Autodesk Inventor part; units mm, degrees
(part 5 of 6)
  line L3785 (22.09, 25.7636) -> (22.09, 26.7636)
  line L3786 (22.09, 26.7636) -> (21.09, 26.7636)
  line L3787 (21.09, 26.7636) -> (21.09, 25.7636)
  line L3788 (21.9917, 25.7636) -> (22.9917, 25.7636)
  line L3789 (22.9917, 25.7636) -> (22.9917, 26.7636)
  line L3790 (22.9917, 26.7636) -> (21.9917, 26.7636)
  line L3791 (21.9917, 26.7636) -> (21.9917, 25.7636)
  line L3792 (12.7334, 25.789) -> (13.7334, 25.789)
  line L3793 (13.7334, 25.789) -> (13.7334, 26.789)
  line L3794 (13.7334, 26.789) -> (12.7334, 26.789)
  line L3795 (12.7334, 26.789) -> (12.7334, 25.789)
  line L3796 (14.4479, 25.789) -> (15.4479, 25.789)
  line L3797 (15.4479, 25.789) -> (15.4479, 26.789)
  line L3798 (15.4479, 26.789) -> (14.4479, 26.789)
  line L3799 (14.4479, 26.789) -> (14.4479, 25.789)
  line L3800 (15.0321, 25.789) -> (16.0321, 25.789)
  line L3801 (16.0321, 25.789) -> (16.0321, 26.789)
  line L3802 (16.0321, 26.789) -> (15.0321, 26.789)
  line L3803 (15.0321, 26.789) -> (15.0321, 25.789)
  line L3804 (19.4517, 25.789) -> (20.4517, 25.789)
  line L3805 (20.4517, 25.789) -> (20.4517, 26.789)
  line L3806 (20.4517, 26.789) -> (19.4517, 26.789)
  line L3807 (19.4517, 26.789) -> (19.4517, 25.789)
  line L3808 (20.3661, 25.789) -> (21.3661, 25.789)
  line L3809 (21.3661, 25.789) -> (21.3661, 26.789)
  line L3810 (21.3661, 26.789) -> (20.3661, 26.789)
  line L3811 (20.3661, 26.789) -> (20.3661, 25.789)
  line L3812 (21.0773, 25.789) -> (22.0773, 25.789)
  line L3813 (22.0773, 25.789) -> (22.0773, 26.789)
  line L3814 (22.0773, 26.789) -> (21.0773, 26.789)
  line L3815 (21.0773, 26.789) -> (21.0773, 25.789)
  line L3816 (22.0171, 25.789) -> (23.0171, 25.789)
  line L3817 (23.0171, 25.789) -> (23.0171, 26.789)
  line L3818 (23.0171, 26.789) -> (22.0171, 26.789)
  line L3819 (22.0171, 26.789) -> (22.0171, 25.789)
  line L3820 (12.7588, 25.8144) -> (13.7588, 25.8144)
  line L3821 (13.7588, 25.8144) -> (13.7588, 26.8144)
  line L3822 (13.7588, 26.8144) -> (12.7588, 26.8144)
  line L3823 (12.7588, 26.8144) -> (12.7588, 25.8144)
  line L3824 (14.4733, 25.8144) -> (15.4733, 25.8144)
  line L3825 (15.4733, 25.8144) -> (15.4733, 26.8144)
  line L3826 (15.4733, 26.8144) -> (14.4733, 26.8144)
  line L3827 (14.4733, 26.8144) -> (14.4733, 25.8144)
  line L3828 (19.4517, 25.8144) -> (20.4517, 25.8144)
  line L3829 (20.4517, 25.8144) -> (20.4517, 26.8144)
  line L3830 (20.4517, 26.8144) -> (19.4517, 26.8144)
  line L3831 (19.4517, 26.8144) -> (19.4517, 25.8144)
  line L3832 (20.3661, 25.8144) -> (21.3661, 25.8144)
  line L3833 (21.3661, 25.8144) -> (21.3661, 26.8144)
  line L3834 (21.3661, 26.8144) -> (20.3661, 26.8144)
  line L3835 (20.3661, 26.8144) -> (20.3661, 25.8144)
  line L3836 (21.0773, 25.8144) -> (22.0773, 25.8144)
  line L3837 (22.0773, 25.8144) -> (22.0773, 26.8144)
  line L3838 (22.0773, 26.8144) -> (21.0773, 26.8144)
  line L3839 (21.0773, 26.8144) -> (21.0773, 25.8144)
  line L3840 (22.0171, 25.8144) -> (23.0171, 25.8144)
  line L3841 (23.0171, 25.8144) -> (23.0171, 26.8144)
  line L3842 (23.0171, 26.8144) -> (22.0171, 26.8144)
  line L3843 (22.0171, 26.8144) -> (22.0171, 25.8144)
  line L3844 (12.7715, 25.8398) -> (13.7715, 25.8398)
  line L3845 (13.7715, 25.8398) -> (13.7715, 26.8398)
  line L3846 (13.7715, 26.8398) -> (12.7715, 26.8398)
  line L3847 (12.7715, 26.8398) -> (12.7715, 25.8398)
  line L3848 (14.4987, 25.8398) -> (15.4987, 25.8398)
  line L3849 (15.4987, 25.8398) -> (15.4987, 26.8398)
  line L3850 (15.4987, 26.8398) -> (14.4987, 26.8398)
  line L3851 (14.4987, 26.8398) -> (14.4987, 25.8398)
  line L3852 (19.4517, 25.8398) -> (20.4517, 25.8398)
  line L3853 (20.4517, 25.8398) -> (20.4517, 26.8398)
  line L3854 (20.4517, 26.8398) -> (19.4517, 26.8398)
  line L3855 (19.4517, 26.8398) -> (19.4517, 25.8398)
  line L3856 (20.3788, 25.8398) -> (21.3788, 25.8398)
  line L3857 (21.3788, 25.8398) -> (21.3788, 26.8398)
  line L3858 (21.3788, 26.8398) -> (20.3788, 26.8398)
  line L3859 (20.3788, 26.8398) -> (20.3788, 25.8398)
  line L3860 (21.0519, 25.8398) -> (22.0519, 25.8398)
  line L3861 (22.0519, 25.8398) -> (22.0519, 26.8398)
  line L3862 (22.0519, 26.8398) -> (21.0519, 26.8398)
  line L3863 (21.0519, 26.8398) -> (21.0519, 25.8398)
  line L3864 (22.0425, 25.8398) -> (23.0425, 25.8398)
  line L3865 (23.0425, 25.8398) -> (23.0425, 26.8398)
  line L3866 (23.0425, 26.8398) -> (22.0425, 26.8398)
  line L3867 (22.0425, 26.8398) -> (22.0425, 25.8398)
  line L3868 (12.7969, 25.8652) -> (13.7969, 25.8652)
  line L3869 (13.7969, 25.8652) -> (13.7969, 26.8652)
  line L3870 (13.7969, 26.8652) -> (12.7969, 26.8652)
  line L3871 (12.7969, 26.8652) -> (12.7969, 25.8652)
  line L3872 (14.5114, 25.8652) -> (15.5114, 25.8652)
  line L3873 (15.5114, 25.8652) -> (15.5114, 26.8652)
  line L3874 (15.5114, 26.8652) -> (14.5114, 26.8652)
  line L3875 (14.5114, 26.8652) -> (14.5114, 25.8652)
  line L3876 (19.439, 25.8652) -> (20.439, 25.8652)
  line L3877 (20.439, 25.8652) -> (20.439, 26.8652)
  line L3878 (20.439, 26.8652) -> (19.439, 26.8652)
  line L3879 (19.439, 26.8652) -> (19.439, 25.8652)
  line L3880 (20.3788, 25.8652) -> (21.3788, 25.8652)
  line L3881 (21.3788, 25.8652) -> (21.3788, 26.8652)
  line L3882 (21.3788, 26.8652) -> (20.3788, 26.8652)
  line L3883 (20.3788, 26.8652) -> (20.3788, 25.8652)
  line L3884 (21.0519, 25.8652) -> (22.0519, 25.8652)
  line L3885 (22.0519, 25.8652) -> (22.0519, 26.8652)
  line L3886 (22.0519, 26.8652) -> (21.0519, 26.8652)
  line L3887 (21.0519, 26.8652) -> (21.0519, 25.8652)
  line L3888 (22.0425, 25.8652) -> (23.0425, 25.8652)
  line L3889 (23.0425, 25.8652) -> (23.0425, 26.8652)
  line L3890 (23.0425, 26.8652) -> (22.0425, 26.8652)
  line L3891 (22.0425, 26.8652) -> (22.0425, 25.8652)
  line L3892 (12.835, 25.8906) -> (13.835, 25.8906)
  line L3893 (13.835, 25.8906) -> (13.835, 26.8906)
  line L3894 (13.835, 26.8906) -> (12.835, 26.8906)
  line L3895 (12.835, 26.8906) -> (12.835, 25.8906)
  line L3896 (14.5368, 25.8906) -> (15.5368, 25.8906)
  line L3897 (15.5368, 25.8906) -> (15.5368, 26.8906)
  line L3898 (15.5368, 26.8906) -> (14.5368, 26.8906)
  line L3899 (14.5368, 26.8906) -> (14.5368, 25.8906)
  line L3900 (19.439, 25.8906) -> (20.439, 25.8906)
  line L3901 (20.439, 25.8906) -> (20.439, 26.8906)
  line L3902 (20.439, 26.8906) -> (19.439, 26.8906)
  line L3903 (19.439, 26.8906) -> (19.439, 25.8906)
  line L3904 (20.3788, 25.8906) -> (21.3788, 25.8906)
  line L3905 (21.3788, 25.8906) -> (21.3788, 26.8906)
  line L3906 (21.3788, 26.8906) -> (20.3788, 26.8906)
  line L3907 (20.3788, 26.8906) -> (20.3788, 25.8906)
  line L3908 (21.0519, 25.8906) -> (22.0519, 25.8906)
  line L3909 (22.0519, 25.8906) -> (22.0519, 26.8906)
  line L3910 (22.0519, 26.8906) -> (21.0519, 26.8906)
  line L3911 (21.0519, 26.8906) -> (21.0519, 25.8906)
  line L3912 (22.0679, 25.8906) -> (23.0679, 25.8906)
  line L3913 (23.0679, 25.8906) -> (23.0679, 26.8906)
  line L3914 (23.0679, 26.8906) -> (22.0679, 26.8906)
  line L3915 (22.0679, 26.8906) -> (22.0679, 25.8906)
  line L3916 (12.8477, 25.916) -> (13.8477, 25.916)
  line L3917 (13.8477, 25.916) -> (13.8477, 26.916)
  line L3918 (13.8477, 26.916) -> (12.8477, 26.916)
  line L3919 (12.8477, 26.916) -> (12.8477, 25.916)
  line L3920 (14.5622, 25.916) -> (15.5622, 25.916)
  line L3921 (15.5622, 25.916) -> (15.5622, 26.916)
  line L3922 (15.5622, 26.916) -> (14.5622, 26.916)
  line L3923 (14.5622, 26.916) -> (14.5622, 25.916)
  line L3924 (19.439, 25.916) -> (20.439, 25.916)
  line L3925 (20.439, 25.916) -> (20.439, 26.916)
  line L3926 (20.439, 26.916) -> (19.439, 26.916)
  line L3927 (19.439, 26.916) -> (19.439, 25.916)
  line L3928 (20.3915, 25.916) -> (21.3915, 25.916)
  line L3929 (21.3915, 25.916) -> (21.3915, 26.916)
  line L3930 (21.3915, 26.916) -> (20.3915, 26.916)
  line L3931 (20.3915, 26.916) -> (20.3915, 25.916)
  line L3932 (21.0392, 25.916) -> (22.0392, 25.916)
  line L3933 (22.0392, 25.916) -> (22.0392, 26.916)
  line L3934 (22.0392, 26.916) -> (21.0392, 26.916)
  line L3935 (21.0392, 26.916) -> (21.0392, 25.916)
  line L3936 (22.0679, 25.916) -> (23.0679, 25.916)
  line L3937 (23.0679, 25.916) -> (23.0679, 26.916)
  line L3938 (23.0679, 26.916) -> (22.0679, 26.916)
  line L3939 (22.0679, 26.916) -> (22.0679, 25.916)
  line L3940 (12.8731, 25.9414) -> (13.8731, 25.9414)
  line L3941 (13.8731, 25.9414) -> (13.8731, 26.9414)
  line L3942 (13.8731, 26.9414) -> (12.8731, 26.9414)
  line L3943 (12.8731, 26.9414) -> (12.8731, 25.9414)
  line L3944 (14.5749, 25.9414) -> (15.5749, 25.9414)
  line L3945 (15.5749, 25.9414) -> (15.5749, 26.9414)
  line L3946 (15.5749, 26.9414) -> (14.5749, 26.9414)
  line L3947 (14.5749, 26.9414) -> (14.5749, 25.9414)
  line L3948 (19.4517, 25.9414) -> (20.4517, 25.9414)
  line L3949 (20.4517, 25.9414) -> (20.4517, 26.9414)
  line L3950 (20.4517, 26.9414) -> (19.4517, 26.9414)
  line L3951 (19.4517, 26.9414) -> (19.4517, 25.9414)
  line L3952 (20.3915, 25.9414) -> (21.3915, 25.9414)
  line L3953 (21.3915, 25.9414) -> (21.3915, 26.9414)
  line L3954 (21.3915, 26.9414) -> (20.3915, 26.9414)
  line L3955 (20.3915, 26.9414) -> (20.3915, 25.9414)
  line L3956 (21.0265, 25.9414) -> (22.0265, 25.9414)
  line L3957 (22.0265, 25.9414) -> (22.0265, 26.9414)
  line L3958 (22.0265, 26.9414) -> (21.0265, 26.9414)
  line L3959 (21.0265, 26.9414) -> (21.0265, 25.9414)
  line L3960 (22.0933, 25.9414) -> (23.0933, 25.9414)
  line L3961 (23.0933, 25.9414) -> (23.0933, 26.9414)
  line L3962 (23.0933, 26.9414) -> (22.0933, 26.9414)
  line L3963 (22.0933, 26.9414) -> (22.0933, 25.9414)
  line L3964 (12.8985, 25.9668) -> (13.8985, 25.9668)
  line L3965 (13.8985, 25.9668) -> (13.8985, 26.9668)
  line L3966 (13.8985, 26.9668) -> (12.8985, 26.9668)
  line L3967 (12.8985, 26.9668) -> (12.8985, 25.9668)
  line L3968 (14.6003, 25.9668) -> (15.6003, 25.9668)
  line L3969 (15.6003, 25.9668) -> (15.6003, 26.9668)
  line L3970 (15.6003, 26.9668) -> (14.6003, 26.9668)
  line L3971 (14.6003, 26.9668) -> (14.6003, 25.9668)
  line L3972 (19.439, 25.9668) -> (20.439, 25.9668)
  line L3973 (20.439, 25.9668) -> (20.439, 26.9668)
  line L3974 (20.439, 26.9668) -> (19.439, 26.9668)
  line L3975 (19.439, 26.9668) -> (19.439, 25.9668)
  line L3976 (20.3915, 25.9668) -> (21.3915, 25.9668)
  line L3977 (21.3915, 25.9668) -> (21.3915, 26.9668)
  line L3978 (21.3915, 26.9668) -> (20.3915, 26.9668)
  line L3979 (20.3915, 26.9668) -> (20.3915, 25.9668)
  line L3980 (21.0265, 25.9668) -> (22.0265, 25.9668)
  line L3981 (22.0265, 25.9668) -> (22.0265, 26.9668)
  line L3982 (22.0265, 26.9668) -> (21.0265, 26.9668)
  line L3983 (21.0265, 26.9668) -> (21.0265, 25.9668)
  line L3984 (22.0933, 25.9668) -> (23.0933, 25.9668)
  line L3985 (23.0933, 25.9668) -> (23.0933, 26.9668)
  line L3986 (23.0933, 26.9668) -> (22.0933, 26.9668)
  line L3987 (22.0933, 26.9668) -> (22.0933, 25.9668)
  line L3988 (12.9366, 25.9922) -> (13.9366, 25.9922)
  line L3989 (13.9366, 25.9922) -> (13.9366, 26.9922)
  line L3990 (13.9366, 26.9922) -> (12.9366, 26.9922)
  line L3991 (12.9366, 26.9922) -> (12.9366, 25.9922)
  line L3992 (14.6257, 25.9922) -> (15.6257, 25.9922)
  line L3993 (15.6257, 25.9922) -> (15.6257, 26.9922)
  line L3994 (15.6257, 26.9922) -> (14.6257, 26.9922)
  line L3995 (14.6257, 26.9922) -> (14.6257, 25.9922)
  line L3996 (19.439, 25.9922) -> (20.439, 25.9922)
  line L3997 (20.439, 25.9922) -> (20.439, 26.9922)
  line L3998 (20.439, 26.9922) -> (19.439, 26.9922)
  line L3999 (19.439, 26.9922) -> (19.439, 25.9922)
  line L4000 (20.4042, 25.9922) -> (21.4042, 25.9922)
  line L4001 (21.4042, 25.9922) -> (21.4042, 26.9922)
  line L4002 (21.4042, 26.9922) -> (20.4042, 26.9922)
  line L4003 (20.4042, 26.9922) -> (20.4042, 25.9922)
  line L4004 (21.0138, 25.9922) -> (22.0138, 25.9922)
  line L4005 (22.0138, 25.9922) -> (22.0138, 26.9922)
  line L4006 (22.0138, 26.9922) -> (21.0138, 26.9922)
  line L4007 (21.0138, 26.9922) -> (21.0138, 25.9922)
  line L4008 (22.106, 25.9922) -> (23.106, 25.9922)
  line L4009 (23.106, 25.9922) -> (23.106, 26.9922)
  line L4010 (23.106, 26.9922) -> (22.106, 26.9922)
  line L4011 (22.106, 26.9922) -> (22.106, 25.9922)
  line L4012 (12.9493, 26.0176) -> (13.9493, 26.0176)
  line L4013 (13.9493, 26.0176) -> (13.9493, 27.0176)
  line L4014 (13.9493, 27.0176) -> (12.9493, 27.0176)
  line L4015 (12.9493, 27.0176) -> (12.9493, 26.0176)
  line L4016 (14.6257, 26.0176) -> (15.6257, 26.0176)
  line L4017 (15.6257, 26.0176) -> (15.6257, 27.0176)
  line L4018 (15.6257, 27.0176) -> (14.6257, 27.0176)
  line L4019 (14.6257, 27.0176) -> (14.6257, 26.0176)
  line L4020 (19.439, 26.0176) -> (20.439, 26.0176)
  line L4021 (20.439, 26.0176) -> (20.439, 27.0176)
  line L4022 (20.439, 27.0176) -> (19.439, 27.0176)
  line L4023 (19.439, 27.0176) -> (19.439, 26.0176)
  line L4024 (20.4042, 26.0176) -> (21.4042, 26.0176)
  line L4025 (21.4042, 26.0176) -> (21.4042, 27.0176)
  line L4026 (21.4042, 27.0176) -> (20.4042, 27.0176)
  line L4027 (20.4042, 27.0176) -> (20.4042, 26.0176)
  line L4028 (21.0011, 26.0176) -> (22.0011, 26.0176)
  line L4029 (22.0011, 26.0176) -> (22.0011, 27.0176)
  line L4030 (22.0011, 27.0176) -> (21.0011, 27.0176)
  line L4031 (21.0011, 27.0176) -> (21.0011, 26.0176)
  line L4032 (22.1187, 26.0176) -> (23.1187, 26.0176)
  line L4033 (23.1187, 26.0176) -> (23.1187, 27.0176)
  line L4034 (23.1187, 27.0176) -> (22.1187, 27.0176)
  line L4035 (22.1187, 27.0176) -> (22.1187, 26.0176)
  line L4036 (12.9747, 26.043) -> (13.9747, 26.043)
  line L4037 (13.9747, 26.043) -> (13.9747, 27.043)
  line L4038 (13.9747, 27.043) -> (12.9747, 27.043)
  line L4039 (12.9747, 27.043) -> (12.9747, 26.043)
  line L4040 (14.5415, 26.5303) -> (14.5669, 26.5303)
  line L4041 (14.5669, 26.5303) -> (14.5669, 26.5557)
  line L4042 (14.5669, 26.5557) -> (14.5415, 26.5557)
  line L4043 (14.5415, 26.5557) -> (14.5415, 26.5303)
  line L4044 (14.6257, 26.043) -> (15.6257, 26.043)
  line L4045 (15.6257, 26.043) -> (15.6257, 27.043)
  line L4046 (15.6257, 27.043) -> (14.6257, 27.043)
  line L4047 (14.6257, 27.043) -> (14.6257, 26.043)
  line L4048 (19.439, 26.043) -> (20.439, 26.043)
  line L4049 (20.439, 26.043) -> (20.439, 27.043)
  line L4050 (20.439, 27.043) -> (19.439, 27.043)
  line L4051 (19.439, 27.043) -> (19.439, 26.043)
  line L4052 (20.4169, 26.043) -> (21.4169, 26.043)
  line L4053 (21.4169, 26.043) -> (21.4169, 27.043)
  line L4054 (21.4169, 27.043) -> (20.4169, 27.043)
  line L4055 (20.4169, 27.043) -> (20.4169, 26.043)
  line L4056 (21.0011, 26.043) -> (22.0011, 26.043)
  line L4057 (22.0011, 26.043) -> (22.0011, 27.043)
  line L4058 (22.0011, 27.043) -> (21.0011, 27.043)
  line L4059 (21.0011, 27.043) -> (21.0011, 26.043)
  line L4060 (22.1314, 26.043) -> (23.1314, 26.043)
  line L4061 (23.1314, 26.043) -> (23.1314, 27.043)
  line L4062 (23.1314, 27.043) -> (22.1314, 27.043)
  line L4063 (22.1314, 27.043) -> (22.1314, 26.043)
  line L4064 (13.0128, 26.0684) -> (14.0128, 26.0684)
  line L4065 (14.0128, 26.0684) -> (14.0128, 27.0684)
  line L4066 (14.0128, 27.0684) -> (13.0128, 27.0684)
  line L4067 (13.0128, 27.0684) -> (13.0128, 26.0684)
  line L4068 (14.0415, 26.0684) -> (15.0415, 26.0684)
  line L4069 (15.0415, 26.0684) -> (15.0415, 27.0684)
  line L4070 (15.0415, 27.0684) -> (14.0415, 27.0684)
  line L4071 (14.0415, 27.0684) -> (14.0415, 26.0684)
  line L4072 (14.6257, 26.0684) -> (15.6257, 26.0684)
  line L4073 (15.6257, 26.0684) -> (15.6257, 27.0684)
  line L4074 (15.6257, 27.0684) -> (14.6257, 27.0684)
  line L4075 (14.6257, 27.0684) -> (14.6257, 26.0684)
  line L4076 (13.0382, 26.0938) -> (14.0382, 26.0938)
  line L4077 (14.0382, 26.0938) -> (14.0382, 27.0938)
  line L4078 (14.0382, 27.0938) -> (13.0382, 27.0938)
  line L4079 (13.0382, 27.0938) -> (13.0382, 26.0938)
  line L4080 (14.0161, 26.0938) -> (15.0161, 26.0938)
  line L4081 (15.0161, 26.0938) -> (15.0161, 27.0938)
  line L4082 (15.0161, 27.0938) -> (14.0161, 27.0938)
  line L4083 (14.0161, 27.0938) -> (14.0161, 26.0938)
  line L4084 (14.613, 26.0938) -> (15.613, 26.0938)
  line L4085 (15.613, 26.0938) -> (15.613, 27.0938)
  line L4086 (15.613, 27.0938) -> (14.613, 27.0938)
  line L4087 (14.613, 27.0938) -> (14.613, 26.0938)
  line L4088 (13.0382, 26.1192) -> (14.0382, 26.1192)
  line L4089 (14.0382, 26.1192) -> (14.0382, 27.1192)
  line L4090 (14.0382, 27.1192) -> (13.0382, 27.1192)
  line L4091 (13.0382, 27.1192) -> (13.0382, 26.1192)
  line L4092 (13.9907, 26.1192) -> (14.9907, 26.1192)
  line L4093 (14.9907, 26.1192) -> (14.9907, 27.1192)
  line L4094 (14.9907, 27.1192) -> (13.9907, 27.1192)
  line L4095 (13.9907, 27.1192) -> (13.9907, 26.1192)
  line L4096 (14.613, 26.1192) -> (15.613, 26.1192)
  line L4097 (15.613, 26.1192) -> (15.613, 27.1192)
  line L4098 (15.613, 27.1192) -> (14.613, 27.1192)
  line L4099 (14.613, 27.1192) -> (14.613, 26.1192)
  line L4100 (13.0255, 26.1446) -> (14.0255, 26.1446)
  line L4101 (14.0255, 26.1446) -> (14.0255, 27.1446)
  line L4102 (14.0255, 27.1446) -> (13.0255, 27.1446)
  line L4103 (13.0255, 27.1446) -> (13.0255, 26.1446)
  line L4104 (13.9653, 26.1446) -> (14.9653, 26.1446)
  line L4105 (14.9653, 26.1446) -> (14.9653, 27.1446)
  line L4106 (14.9653, 27.1446) -> (13.9653, 27.1446)
  line L4107 (13.9653, 27.1446) -> (13.9653, 26.1446)
  line L4108 (14.613, 26.1446) -> (15.613, 26.1446)
  line L4109 (15.613, 26.1446) -> (15.613, 27.1446)
  line L4110 (15.613, 27.1446) -> (14.613, 27.1446)
  line L4111 (14.613, 27.1446) -> (14.613, 26.1446)
  line L4112 (13.0128, 26.17) -> (14.0128, 26.17)
  line L4113 (14.0128, 26.17) -> (14.0128, 27.17)
  line L4114 (14.0128, 27.17) -> (13.0128, 27.17)
  line L4115 (13.0128, 27.17) -> (13.0128, 26.17)
  line L4116 (13.9526, 26.17) -> (14.9526, 26.17)
  line L4117 (14.9526, 26.17) -> (14.9526, 27.17)
  line L4118 (14.9526, 27.17) -> (13.9526, 27.17)
  line L4119 (13.9526, 27.17) -> (13.9526, 26.17)
  line L4120 (14.6003, 26.17) -> (15.6003, 26.17)
  line L4121 (15.6003, 26.17) -> (15.6003, 27.17)
  line L4122 (15.6003, 27.17) -> (14.6003, 27.17)
  line L4123 (14.6003, 27.17) -> (14.6003, 26.17)
  line L4124 (13.0001, 26.1954) -> (14.0001, 26.1954)
  line L4125 (14.0001, 26.1954) -> (14.0001, 27.1954)
  line L4126 (14.0001, 27.1954) -> (13.0001, 27.1954)
  line L4127 (13.0001, 27.1954) -> (13.0001, 26.1954)
  line L4128 (13.9272, 26.1954) -> (14.9272, 26.1954)
  line L4129 (14.9272, 26.1954) -> (14.9272, 27.1954)
  line L4130 (14.9272, 27.1954) -> (13.9272, 27.1954)
  line L4131 (13.9272, 27.1954) -> (13.9272, 26.1954)
  line L4132 (14.6003, 26.1954) -> (15.6003, 26.1954)
  line L4133 (15.6003, 26.1954) -> (15.6003, 27.1954)
  line L4134 (15.6003, 27.1954) -> (14.6003, 27.1954)
  line L4135 (14.6003, 27.1954) -> (14.6003, 26.1954)
  line L4136 (12.9747, 26.2208) -> (13.9747, 26.2208)
  line L4137 (13.9747, 26.2208) -> (13.9747, 27.2208)
  line L4138 (13.9747, 27.2208) -> (12.9747, 27.2208)
  line L4139 (12.9747, 27.2208) -> (12.9747, 26.2208)
  line L4140 (13.9018, 26.2208) -> (14.9018, 26.2208)
  line L4141 (14.9018, 26.2208) -> (14.9018, 27.2208)
  line L4142 (14.9018, 27.2208) -> (13.9018, 27.2208)
  line L4143 (13.9018, 27.2208) -> (13.9018, 26.2208)
  line L4144 (14.5876, 26.2208) -> (15.5876, 26.2208)
  line L4145 (15.5876, 26.2208) -> (15.5876, 27.2208)
  line L4146 (15.5876, 27.2208) -> (14.5876, 27.2208)
  line L4147 (14.5876, 27.2208) -> (14.5876, 26.2208)
  line L4148 (12.9747, 26.2462) -> (13.9747, 26.2462)
  line L4149 (13.9747, 26.2462) -> (13.9747, 27.2462)
  line L4150 (13.9747, 27.2462) -> (12.9747, 27.2462)
  line L4151 (12.9747, 27.2462) -> (12.9747, 26.2462)
  line L4152 (13.8891, 26.2462) -> (14.8891, 26.2462)
  line L4153 (14.8891, 26.2462) -> (14.8891, 27.2462)
  line L4154 (14.8891, 27.2462) -> (13.8891, 27.2462)
  line L4155 (13.8891, 27.2462) -> (13.8891, 26.2462)
  line L4156 (14.5876, 26.2462) -> (15.5876, 26.2462)
  line L4157 (15.5876, 26.2462) -> (15.5876, 27.2462)
  line L4158 (15.5876, 27.2462) -> (14.5876, 27.2462)
  line L4159 (14.5876, 27.2462) -> (14.5876, 26.2462)
  line L4160 (12.9493, 26.2716) -> (13.9493, 26.2716)
  line L4161 (13.9493, 26.2716) -> (13.9493, 27.2716)
  line L4162 (13.9493, 27.2716) -> (12.9493, 27.2716)
  line L4163 (12.9493, 27.2716) -> (12.9493, 26.2716)
  line L4164 (13.8637, 26.2716) -> (14.8637, 26.2716)
  line L4165 (14.8637, 26.2716) -> (14.8637, 27.2716)
  line L4166 (14.8637, 27.2716) -> (13.8637, 27.2716)
  line L4167 (13.8637, 27.2716) -> (13.8637, 26.2716)
  line L4168 (14.5749, 26.2716) -> (15.5749, 26.2716)
  line L4169 (15.5749, 26.2716) -> (15.5749, 27.2716)
  line L4170 (15.5749, 27.2716) -> (14.5749, 27.2716)
  line L4171 (14.5749, 27.2716) -> (14.5749, 26.2716)
  line L4172 (12.9366, 26.297) -> (13.9366, 26.297)
  line L4173 (13.9366, 26.297) -> (13.9366, 27.297)
  line L4174 (13.9366, 27.297) -> (12.9366, 27.297)
  line L4175 (12.9366, 27.297) -> (12.9366, 26.297)
  line L4176 (13.8383, 26.297) -> (14.8383, 26.297)
  line L4177 (14.8383, 26.297) -> (14.8383, 27.297)
  line L4178 (14.8383, 27.297) -> (13.8383, 27.297)
  line L4179 (13.8383, 27.297) -> (13.8383, 26.297)
  line L4180 (14.5749, 26.297) -> (15.5749, 26.297)
  line L4181 (15.5749, 26.297) -> (15.5749, 27.297)
  line L4182 (15.5749, 27.297) -> (14.5749, 27.297)
  line L4183 (14.5749, 27.297) -> (14.5749, 26.297)
  line L4184 (12.9112, 26.3224) -> (13.9112, 26.3224)
  line L4185 (13.9112, 26.3224) -> (13.9112, 27.3224)
  line L4186 (13.9112, 27.3224) -> (12.9112, 27.3224)
  line L4187 (12.9112, 27.3224) -> (12.9112, 26.3224)
  line L4188 (13.8129, 26.3224) -> (14.8129, 26.3224)
  line L4189 (14.8129, 26.3224) -> (14.8129, 27.3224)
  line L4190 (14.8129, 27.3224) -> (13.8129, 27.3224)
  line L4191 (13.8129, 27.3224) -> (13.8129, 26.3224)
  line L4192 (14.5622, 26.3224) -> (15.5622, 26.3224)
  line L4193 (15.5622, 26.3224) -> (15.5622, 27.3224)
  line L4194 (15.5622, 27.3224) -> (14.5622, 27.3224)
  line L4195 (14.5622, 27.3224) -> (14.5622, 26.3224)
  line L4196 (12.9112, 26.3478) -> (13.9112, 26.3478)
  line L4197 (13.9112, 26.3478) -> (13.9112, 27.3478)
  line L4198 (13.9112, 27.3478) -> (12.9112, 27.3478)
  line L4199 (12.9112, 27.3478) -> (12.9112, 26.3478)
  line L4200 (13.8002, 26.3478) -> (14.8002, 26.3478)
  line L4201 (14.8002, 26.3478) -> (14.8002, 27.3478)
  line L4202 (14.8002, 27.3478) -> (13.8002, 27.3478)
  line L4203 (13.8002, 27.3478) -> (13.8002, 26.3478)
  line L4204 (14.5622, 26.3478) -> (15.5622, 26.3478)
  line L4205 (15.5622, 26.3478) -> (15.5622, 27.3478)
  line L4206 (15.5622, 27.3478) -> (14.5622, 27.3478)
  line L4207 (14.5622, 27.3478) -> (14.5622, 26.3478)
  line L4208 (12.8858, 26.3732) -> (13.8858, 26.3732)
  line L4209 (13.8858, 26.3732) -> (13.8858, 27.3732)
  line L4210 (13.8858, 27.3732) -> (12.8858, 27.3732)
  line L4211 (12.8858, 27.3732) -> (12.8858, 26.3732)
  line L4212 (13.7748, 26.3732) -> (14.7748, 26.3732)
  line L4213 (14.7748, 26.3732) -> (14.7748, 27.3732)
  line L4214 (14.7748, 27.3732) -> (13.7748, 27.3732)
  line L4215 (13.7748, 27.3732) -> (13.7748, 26.3732)
  line L4216 (14.5495, 26.3732) -> (15.5495, 26.3732)
  line L4217 (15.5495, 26.3732) -> (15.5495, 27.3732)
  line L4218 (15.5495, 27.3732) -> (14.5495, 27.3732)
  line L4219 (14.5495, 27.3732) -> (14.5495, 26.3732)
  line L4220 (12.8731, 26.3986) -> (13.8731, 26.3986)
  line L4221 (13.8731, 26.3986) -> (13.8731, 27.3986)
  line L4222 (13.8731, 27.3986) -> (12.8731, 27.3986)
  line L4223 (12.8731, 27.3986) -> (12.8731, 26.3986)
  line L4224 (13.7494, 26.3986) -> (14.7494, 26.3986)
  line L4225 (14.7494, 26.3986) -> (14.7494, 27.3986)
  line L4226 (14.7494, 27.3986) -> (13.7494, 27.3986)
  line L4227 (13.7494, 27.3986) -> (13.7494, 26.3986)
  line L4228 (14.5368, 26.3986) -> (15.5368, 26.3986)
  line L4229 (15.5368, 26.3986) -> (15.5368, 27.3986)
  line L4230 (15.5368, 27.3986) -> (14.5368, 27.3986)
  line L4231 (14.5368, 27.3986) -> (14.5368, 26.3986)
  line L4232 (12.8731, 26.424) -> (13.8731, 26.424)
  line L4233 (13.8731, 26.424) -> (13.8731, 27.424)
  line L4234 (13.8731, 27.424) -> (12.8731, 27.424)
  line L4235 (12.8731, 27.424) -> (12.8731, 26.424)
  line L4236 (13.724, 26.424) -> (14.724, 26.424)
  line L4237 (14.724, 26.424) -> (14.724, 27.424)
  line L4238 (14.724, 27.424) -> (13.724, 27.424)
  line L4239 (13.724, 27.424) -> (13.724, 26.424)
  line L4240 (14.5368, 26.424) -> (15.5368, 26.424)
  line L4241 (15.5368, 26.424) -> (15.5368, 27.424)
  line L4242 (15.5368, 27.424) -> (14.5368, 27.424)
  line L4243 (14.5368, 27.424) -> (14.5368, 26.424)
  line L4244 (12.8604, 26.4494) -> (13.8604, 26.4494)
  line L4245 (13.8604, 26.4494) -> (13.8604, 27.4494)
  line L4246 (13.8604, 27.4494) -> (12.8604, 27.4494)
  line L4247 (12.8604, 27.4494) -> (12.8604, 26.4494)
  line L4248 (13.7113, 26.4494) -> (14.7113, 26.4494)
  line L4249 (14.7113, 26.4494) -> (14.7113, 27.4494)
  line L4250 (14.7113, 27.4494) -> (13.7113, 27.4494)
  line L4251 (13.7113, 27.4494) -> (13.7113, 26.4494)
  line L4252 (14.5241, 26.4494) -> (15.5241, 26.4494)
  line L4253 (15.5241, 26.4494) -> (15.5241, 27.4494)
  line L4254 (15.5241, 27.4494) -> (14.5241, 27.4494)
  line L4255 (14.5241, 27.4494) -> (14.5241, 26.4494)
  line L4256 (12.835, 26.4748) -> (13.835, 26.4748)
  line L4257 (13.835, 26.4748) -> (13.835, 27.4748)
  line L4258 (13.835, 27.4748) -> (12.835, 27.4748)
  line L4259 (12.835, 27.4748) -> (12.835, 26.4748)
  line L4260 (13.6859, 26.4748) -> (14.6859, 26.4748)
  line L4261 (14.6859, 26.4748) -> (14.6859, 27.4748)
  line L4262 (14.6859, 27.4748) -> (13.6859, 27.4748)
  line L4263 (13.6859, 27.4748) -> (13.6859, 26.4748)
  line L4264 (14.5114, 26.4748) -> (15.5114, 26.4748)
  line L4265 (15.5114, 26.4748) -> (15.5114, 27.4748)
  line L4266 (15.5114, 27.4748) -> (14.5114, 27.4748)
  line L4267 (14.5114, 27.4748) -> (14.5114, 26.4748)
  line L4268 (12.8223, 26.5002) -> (13.8223, 26.5002)
  line L4269 (13.8223, 26.5002) -> (13.8223, 27.5002)
  line L4270 (13.8223, 27.5002) -> (12.8223, 27.5002)
  line L4271 (12.8223, 27.5002) -> (12.8223, 26.5002)
  line L4272 (13.6605, 26.5002) -> (14.6605, 26.5002)
  line L4273 (14.6605, 26.5002) -> (14.6605, 27.5002)
  line L4274 (14.6605, 27.5002) -> (13.6605, 27.5002)
  line L4275 (13.6605, 27.5002) -> (13.6605, 26.5002)
  line L4276 (14.4987, 26.5002) -> (15.4987, 26.5002)
  line L4277 (15.4987, 26.5002) -> (15.4987, 27.5002)
  line L4278 (15.4987, 27.5002) -> (14.4987, 27.5002)
  line L4279 (14.4987, 27.5002) -> (14.4987, 26.5002)
  line L4280 (12.8223, 26.5256) -> (13.8223, 26.5256)
  line L4281 (13.8223, 26.5256) -> (13.8223, 27.5256)
  line L4282 (13.8223, 27.5256) -> (12.8223, 27.5256)
  line L4283 (12.8223, 27.5256) -> (12.8223, 26.5256)
  line L4284 (13.6478, 26.5256) -> (14.6478, 26.5256)
  line L4285 (14.6478, 26.5256) -> (14.6478, 27.5256)
  line L4286 (14.6478, 27.5256) -> (13.6478, 27.5256)
  line L4287 (13.6478, 27.5256) -> (13.6478, 26.5256)
  line L4288 (14.486, 26.5256) -> (15.486, 26.5256)
  line L4289 (15.486, 26.5256) -> (15.486, 27.5256)
  line L4290 (15.486, 27.5256) -> (14.486, 27.5256)
  line L4291 (14.486, 27.5256) -> (14.486, 26.5256)
  line L4292 (13.2969, 27.0383) -> (13.3223, 27.0383)
  line L4293 (13.3223, 27.0383) -> (13.3223, 27.0637)
  line L4294 (13.3223, 27.0637) -> (13.2969, 27.0637)
  line L4295 (13.2969, 27.0637) -> (13.2969, 27.0383)
  line L4296 (13.6224, 26.551) -> (14.6224, 26.551)
  line L4297 (14.6224, 26.551) -> (14.6224, 27.551)
  line L4298 (14.6224, 27.551) -> (13.6224, 27.551)
  line L4299 (13.6224, 27.551) -> (13.6224, 26.551)
  line L4300 (14.4733, 26.551) -> (15.4733, 26.551)
  line L4301 (15.4733, 26.551) -> (15.4733, 27.551)
  line L4302 (15.4733, 27.551) -> (14.4733, 27.551)
  line L4303 (14.4733, 27.551) -> (14.4733, 26.551)
  line L4304 (13.597, 26.5764) -> (14.597, 26.5764)
  line L4305 (14.597, 26.5764) -> (14.597, 27.5764)
  line L4306 (14.597, 27.5764) -> (13.597, 27.5764)
  line L4307 (13.597, 27.5764) -> (13.597, 26.5764)
  line L4308 (14.4606, 26.5764) -> (15.4606, 26.5764)
  line L4309 (15.4606, 26.5764) -> (15.4606, 27.5764)
  line L4310 (15.4606, 27.5764) -> (14.4606, 27.5764)
  line L4311 (14.4606, 27.5764) -> (14.4606, 26.5764)
  line L4312 (13.5716, 26.6018) -> (14.5716, 26.6018)
  line L4313 (14.5716, 26.6018) -> (14.5716, 27.6018)
  line L4314 (14.5716, 27.6018) -> (13.5716, 27.6018)
  line L4315 (13.5716, 27.6018) -> (13.5716, 26.6018)
  line L4316 (14.4479, 26.6018) -> (15.4479, 26.6018)
  line L4317 (15.4479, 26.6018) -> (15.4479, 27.6018)
  line L4318 (15.4479, 27.6018) -> (14.4479, 27.6018)
  line L4319 (14.4479, 27.6018) -> (14.4479, 26.6018)
  line L4320 (13.5589, 26.6272) -> (14.5589, 26.6272)
  line L4321 (14.5589, 26.6272) -> (14.5589, 27.6272)
  line L4322 (14.5589, 27.6272) -> (13.5589, 27.6272)
  line L4323 (13.5589, 27.6272) -> (13.5589, 26.6272)
  line L4324 (14.4352, 26.6272) -> (15.4352, 26.6272)
  line L4325 (15.4352, 26.6272) -> (15.4352, 27.6272)
  line L4326 (15.4352, 27.6272) -> (14.4352, 27.6272)
  line L4327 (14.4352, 27.6272) -> (14.4352, 26.6272)
  line L4328 (13.5335, 26.6526) -> (14.5335, 26.6526)
  line L4329 (14.5335, 26.6526) -> (14.5335, 27.6526)
  line L4330 (14.5335, 27.6526) -> (13.5335, 27.6526)
  line L4331 (13.5335, 27.6526) -> (13.5335, 26.6526)
  line L4332 (14.4225, 26.6526) -> (15.4225, 26.6526)
  line L4333 (15.4225, 26.6526) -> (15.4225, 27.6526)
  line L4334 (15.4225, 27.6526) -> (14.4225, 27.6526)
  line L4335 (14.4225, 27.6526) -> (14.4225, 26.6526)
  line L4336 (13.5081, 26.678) -> (14.5081, 26.678)
  line L4337 (14.5081, 26.678) -> (14.5081, 27.678)
  line L4338 (14.5081, 27.678) -> (13.5081, 27.678)
  line L4339 (13.5081, 27.678) -> (13.5081, 26.678)
  line L4340 (14.4098, 26.678) -> (15.4098, 26.678)
  line L4341 (15.4098, 26.678) -> (15.4098, 27.678)
  line L4342 (15.4098, 27.678) -> (14.4098, 27.678)
  line L4343 (14.4098, 27.678) -> (14.4098, 26.678)
  line L4344 (13.5208, 26.7034) -> (14.5208, 26.7034)
  line L4345 (14.5208, 26.7034) -> (14.5208, 27.7034)
  line L4346 (14.5208, 27.7034) -> (13.5208, 27.7034)
  line L4347 (13.5208, 27.7034) -> (13.5208, 26.7034)
  line L4348 (14.3971, 26.7034) -> (15.3971, 26.7034)
  line L4349 (15.3971, 26.7034) -> (15.3971, 27.7034)
  line L4350 (15.3971, 27.7034) -> (14.3971, 27.7034)
  line L4351 (14.3971, 27.7034) -> (14.3971, 26.7034)
  line L4352 (13.5335, 26.7288) -> (14.5335, 26.7288)
  line L4353 (14.5335, 26.7288) -> (14.5335, 27.7288)
  line L4354 (14.5335, 27.7288) -> (13.5335, 27.7288)
  line L4355 (13.5335, 27.7288) -> (13.5335, 26.7288)
  line L4356 (14.3717, 26.7288) -> (15.3717, 26.7288)
  line L4357 (15.3717, 26.7288) -> (15.3717, 27.7288)
  line L4358 (15.3717, 27.7288) -> (14.3717, 27.7288)
  line L4359 (14.3717, 27.7288) -> (14.3717, 26.7288)
  line L4360 (13.5589, 26.7542) -> (14.5589, 26.7542)
  line L4361 (14.5589, 26.7542) -> (14.5589, 27.7542)
  line L4362 (14.5589, 27.7542) -> (13.5589, 27.7542)
  line L4363 (13.5589, 27.7542) -> (13.5589, 26.7542)
  line L4364 (14.359, 26.7542) -> (15.359, 26.7542)
  line L4365 (15.359, 26.7542) -> (15.359, 27.7542)
  line L4366 (15.359, 27.7542) -> (14.359, 27.7542)
  line L4367 (14.359, 27.7542) -> (14.359, 26.7542)
  line L4368 (13.5716, 26.7796) -> (14.5716, 26.7796)
  line L4369 (14.5716, 26.7796) -> (14.5716, 27.7796)
  line L4370 (14.5716, 27.7796) -> (13.5716, 27.7796)
  line L4371 (13.5716, 27.7796) -> (13.5716, 26.7796)
  line L4372 (14.3336, 26.7796) -> (15.3336, 26.7796)
  line L4373 (15.3336, 26.7796) -> (15.3336, 27.7796)
  line L4374 (15.3336, 27.7796) -> (14.3336, 27.7796)
  line L4375 (14.3336, 27.7796) -> (14.3336, 26.7796)
  line L4376 (13.597, 26.805) -> (14.597, 26.805)
  line L4377 (14.597, 26.805) -> (14.597, 27.805)
  line L4378 (14.597, 27.805) -> (13.597, 27.805)
  line L4379 (13.597, 27.805) -> (13.597, 26.805)
  line L4380 (14.3082, 26.805) -> (15.3082, 26.805)
  line L4381 (15.3082, 26.805) -> (15.3082, 27.805)
  line L4382 (15.3082, 27.805) -> (14.3082, 27.805)
  line L4383 (14.3082, 27.805) -> (14.3082, 26.805)
  line L4384 (13.6224, 26.8304) -> (14.6224, 26.8304)
  line L4385 (14.6224, 26.8304) -> (14.6224, 27.8304)
  line L4386 (14.6224, 27.8304) -> (13.6224, 27.8304)
  line L4387 (13.6224, 27.8304) -> (13.6224, 26.8304)
  line L4388 (14.2828, 26.8304) -> (15.2828, 26.8304)
  line L4389 (15.2828, 26.8304) -> (15.2828, 27.8304)
  line L4390 (15.2828, 27.8304) -> (14.2828, 27.8304)
  line L4391 (14.2828, 27.8304) -> (14.2828, 26.8304)
  line L4392 (13.6478, 26.8558) -> (14.6478, 26.8558)
  line L4393 (14.6478, 26.8558) -> (14.6478, 27.8558)
  line L4394 (14.6478, 27.8558) -> (13.6478, 27.8558)
  line L4395 (13.6478, 27.8558) -> (13.6478, 26.8558)
  line L4396 (14.7447, 27.3431) -> (14.7701, 27.3431)
  line L4397 (14.7701, 27.3431) -> (14.7701, 27.3685)
  line L4398 (14.7701, 27.3685) -> (14.7447, 27.3685)
  line L4399 (14.7447, 27.3685) -> (14.7447, 27.3431)
  line L4400 (13.6859, 26.8812) -> (14.6859, 26.8812)
  line L4401 (14.6859, 26.8812) -> (14.6859, 27.8812)
  line L4402 (14.6859, 27.8812) -> (13.6859, 27.8812)
  line L4403 (13.6859, 27.8812) -> (13.6859, 26.8812)
  line L4404 (13.724, 26.9066) -> (14.724, 26.9066)
  line L4405 (14.724, 26.9066) -> (14.724, 27.9066)
  line L4406 (14.724, 27.9066) -> (13.724, 27.9066)
  line L4407 (13.724, 27.9066) -> (13.724, 26.9066)
  line L4408 (13.7621, 26.932) -> (14.7621, 26.932)
  line L4409 (14.7621, 26.932) -> (14.7621, 27.932)
  line L4410 (14.7621, 27.932) -> (13.7621, 27.932)
  line L4411 (13.7621, 27.932) -> (13.7621, 26.932)
  line L4412 (13.7621, 26.9574) -> (14.7621, 26.9574)
  line L4413 (14.7621, 26.9574) -> (14.7621, 27.9574)
  line L4414 (14.7621, 27.9574) -> (13.7621, 27.9574)
  line L4415 (13.7621, 27.9574) -> (13.7621, 26.9574)
  line L4416 (9.56, 21.883) -> (10.56, 21.883)
  line L4417 (10.56, 21.883) -> (10.56, 22.883)
  line L4418 (10.56, 22.883) -> (9.56, 22.883)
  line L4419 (9.56, 22.883) -> (9.56, 21.883)
  line L4420 (9.56, 21.383) -> (10.56, 21.383)
  line L4421 (10.56, 21.383) -> (10.56, 22.383)
  line L4422 (10.56, 22.383) -> (9.56, 22.383)
  line L4423 (9.56, 22.383) -> (9.56, 21.383)
  line L4424 (9.56, 20.883) -> (10.56, 20.883)
  line L4425 (10.56, 20.883) -> (10.56, 21.883)
  line L4426 (10.56, 21.883) -> (9.56, 21.883)
  line L4427 (9.56, 21.883) -> (9.56, 20.883)
  line L4428 (9.56, 20.383) -> (10.56, 20.383)
  line L4429 (10.56, 20.383) -> (10.56, 21.383)
  line L4430 (10.56, 21.383) -> (9.56, 21.383)
  line L4431 (9.56, 21.383) -> (9.56, 20.383)
  line L4432 (9.56, 19.883) -> (10.56, 19.883)
  line L4433 (10.56, 19.883) -> (10.56, 20.883)
  line L4434 (10.56, 20.883) -> (9.56, 20.883)
  line L4435 (9.56, 20.883) -> (9.56, 19.883)
  line L4436 (9.56, 19.383) -> (10.56, 19.383)
  line L4437 (10.56, 19.383) -> (10.56, 20.383)
  line L4438 (10.56, 20.383) -> (9.56, 20.383)
  line L4439 (9.56, 20.383) -> (9.56, 19.383)
  line L4440 (9.56, 18.883) -> (10.56, 18.883)
  line L4441 (10.56, 18.883) -> (10.56, 19.883)
  line L4442 (10.56, 19.883) -> (9.56, 19.883)
  line L4443 (9.56, 19.883) -> (9.56, 18.883)
  line L4444 (9.56, 18.383) -> (10.56, 18.383)
  line L4445 (10.56, 18.383) -> (10.56, 19.383)
  line L4446 (10.56, 19.383) -> (9.56, 19.383)
  line L4447 (9.56, 19.383) -> (9.56, 18.383)
  line L4448 (9.56, 17.883) -> (10.56, 17.883)
  line L4449 (10.56, 17.883) -> (10.56, 18.883)
  line L4450 (10.56, 18.883) -> (9.56, 18.883)
  line L4451 (9.56, 18.883) -> (9.56, 17.883)
  line L4452 (9.56, 17.383) -> (10.56, 17.383)
  line L4453 (10.56, 17.383) -> (10.56, 18.383)
  line L4454 (10.56, 18.383) -> (9.56, 18.383)
  line L4455 (9.56, 18.383) -> (9.56, 17.383)
  line L4456 (9.56, 16.883) -> (10.56, 16.883)
  line L4457 (10.56, 16.883) -> (10.56, 17.883)
  line L4458 (10.56, 17.883) -> (9.56, 17.883)
  line L4459 (9.56, 17.883) -> (9.56, 16.883)
  line L4460 (9.56, 16.383) -> (10.56, 16.383)
  line L4461 (10.56, 16.383) -> (10.56, 17.383)
  line L4462 (10.56, 17.383) -> (9.56, 17.383)
  line L4463 (9.56, 17.383) -> (9.56, 16.383)
  line L4464 (9.56, 15.883) -> (10.56, 15.883)
  line L4465 (10.56, 15.883) -> (10.56, 16.883)
  line L4466 (10.56, 16.883) -> (9.56, 16.883)
  line L4467 (9.56, 16.883) -> (9.56, 15.883)
  line L4468 (9.56, 15.383) -> (10.56, 15.383)
  line L4469 (10.56, 15.383) -> (10.56, 16.383)
  line L4470 (10.56, 16.383) -> (9.56, 16.383)
  line L4471 (9.56, 16.383) -> (9.56, 15.383)
  line L4472 (9.56, 14.883) -> (10.56, 14.883)
  line L4473 (10.56, 14.883) -> (10.56, 15.883)
  line L4474 (10.56, 15.883) -> (9.56, 15.883)
  line L4475 (9.56, 15.883) -> (9.56, 14.883)
  line L4476 (9.56, 14.383) -> (10.56, 14.383)
  line L4477 (10.56, 14.383) -> (10.56, 15.383)
  line L4478 (10.56, 15.383) -> (9.56, 15.383)
  line L4479 (9.56, 15.383) -> (9.56, 14.383)
  line L4480 (9.56, 13.883) -> (10.56, 13.883)
  line L4481 (10.56, 13.883) -> (10.56, 14.883)
  line L4482 (10.56, 14.883) -> (9.56, 14.883)
  line L4483 (9.56, 14.883) -> (9.56, 13.883)
  line L4484 (9.56, 13.383) -> (10.56, 13.383)
  line L4485 (10.56, 13.383) -> (10.56, 14.383)
  line L4486 (10.56, 14.383) -> (9.56, 14.383)
  line L4487 (9.56, 14.383) -> (9.56, 13.383)
  line L4488 (9.56, 12.883) -> (10.56, 12.883)
  line L4489 (10.56, 12.883) -> (10.56, 13.883)
  line L4490 (10.56, 13.883) -> (9.56, 13.883)
  line L4491 (9.56, 13.883) -> (9.56, 12.883)
  line L4492 (9.56, 12.383) -> (10.56, 12.383)
  line L4493 (10.56, 12.383) -> (10.56, 13.383)
  line L4494 (10.56, 13.383) -> (9.56, 13.383)
  line L4495 (9.56, 13.383) -> (9.56, 12.383)
  line L4496 (9.56, 11.883) -> (10.56, 11.883)
  line L4497 (10.56, 11.883) -> (10.56, 12.883)
  line L4498 (10.56, 12.883) -> (9.56, 12.883)
  line L4499 (9.56, 12.883) -> (9.56, 11.883)
  line L4500 (9.56, 11.383) -> (10.56, 11.383)
  line L4501 (10.56, 11.383) -> (10.56, 12.383)
  line L4502 (10.56, 12.383) -> (9.56, 12.383)
  line L4503 (9.56, 12.383) -> (9.56, 11.383)
  line L4504 (9.56, 10.883) -> (10.56, 10.883)
  line L4505 (10.56, 10.883) -> (10.56, 11.883)
  line L4506 (10.56, 11.883) -> (9.56, 11.883)
  line L4507 (9.56, 11.883) -> (9.56, 10.883)
  line L4508 (9.56, 10.383) -> (10.56, 10.383)
  line L4509 (10.56, 10.383) -> (10.56, 11.383)
  line L4510 (10.56, 11.383) -> (9.56, 11.383)
  line L4511 (9.56, 11.383) -> (9.56, 10.383)
  line L4512 (9.56, 9.883) -> (10.56, 9.883)
  line L4513 (10.56, 9.883) -> (10.56, 10.883)
  line L4514 (10.56, 10.883) -> (9.56, 10.883)
  line L4515 (9.56, 10.883) -> (9.56, 9.883)
  line L4516 (11.28, 8.163) -> (12.28, 8.163)
  line L4517 (12.28, 8.163) -> (12.28, 9.163)
  line L4518 (12.28, 9.163) -> (11.28, 9.163)
  line L4519 (11.28, 9.163) -> (11.28, 8.163)
  line L4520 (11.78, 8.163) -> (12.78, 8.163)
  line L4521 (12.78, 8.163) -> (12.78, 9.163)
  line L4522 (12.78, 9.163) -> (11.78, 9.163)
  line L4523 (11.78, 9.163) -> (11.78, 8.163)
  line L4524 (12.28, 8.163) -> (13.28, 8.163)
  line L4525 (13.28, 8.163) -> (13.28, 9.163)
  line L4526 (13.28, 9.163) -> (12.28, 9.163)
  line L4527 (12.28, 9.163) -> (12.28, 8.163)
  line L4528 (12.78, 8.163) -> (13.78, 8.163)
  line L4529 (13.78, 8.163) -> (13.78, 9.163)
  line L4530 (13.78, 9.163) -> (12.78, 9.163)
  line L4531 (12.78, 9.163) -> (12.78, 8.163)
  line L4532 (13.28, 8.163) -> (14.28, 8.163)
  line L4533 (14.28, 8.163) -> (14.28, 9.163)
  line L4534 (14.28, 9.163) -> (13.28, 9.163)
  line L4535 (13.28, 9.163) -> (13.28, 8.163)
  line L4536 (13.78, 8.163) -> (14.78, 8.163)
  line L4537 (14.78, 8.163) -> (14.78, 9.163)
  line L4538 (14.78, 9.163) -> (13.78, 9.163)
  line L4539 (13.78, 9.163) -> (13.78, 8.163)
  line L4540 (14.28, 8.163) -> (15.28, 8.163)
  line L4541 (15.28, 8.163) -> (15.28, 9.163)
  line L4542 (15.28, 9.163) -> (14.28, 9.163)
  line L4543 (14.28, 9.163) -> (14.28, 8.163)
  line L4544 (14.78, 8.163) -> (15.78, 8.163)
  line L4545 (15.78, 8.163) -> (15.78, 9.163)
  line L4546 (15.78, 9.163) -> (14.78, 9.163)
  line L4547 (14.78, 9.163) -> (14.78, 8.163)
  line L4548 (15.28, 8.163) -> (16.28, 8.163)
  line L4549 (16.28, 8.163) -> (16.28, 9.163)
  line L4550 (16.28, 9.163) -> (15.28, 9.163)
  line L4551 (15.28, 9.163) -> (15.28, 8.163)
  line L4552 (15.78, 8.163) -> (16.78, 8.163)
  line L4553 (16.78, 8.163) -> (16.78, 9.163)
  line L4554 (16.78, 9.163) -> (15.78, 9.163)
  line L4555 (15.78, 9.163) -> (15.78, 8.163)
  line L4556 (16.28, 8.163) -> (17.28, 8.163)
  line L4557 (17.28, 8.163) -> (17.28, 9.163)
  line L4558 (17.28, 9.163) -> (16.28, 9.163)
  line L4559 (16.28, 9.163) -> (16.28, 8.163)
  line L4560 (16.78, 8.163) -> (17.78, 8.163)
  line L4561 (17.78, 8.163) -> (17.78, 9.163)
  line L4562 (17.78, 9.163) -> (16.78, 9.163)
  line L4563 (16.78, 9.163) -> (16.78, 8.163)
  line L4564 (17.28, 8.163) -> (18.28, 8.163)
  line L4565 (18.28, 8.163) -> (18.28, 9.163)
  line L4566 (18.28, 9.163) -> (17.28, 9.163)
  line L4567 (17.28, 9.163) -> (17.28, 8.163)
  line L4568 (17.78, 8.163) -> (18.78, 8.163)
  line L4569 (18.78, 8.163) -> (18.78, 9.163)
  line L4570 (18.78, 9.163) -> (17.78, 9.163)
  line L4571 (17.78, 9.163) -> (17.78, 8.163)
  line L4572 (18.28, 8.163) -> (19.28, 8.163)
  line L4573 (19.28, 8.163) -> (19.28, 9.163)
  line L4574 (19.28, 9.163) -> (18.28, 9.163)
  line L4575 (18.28, 9.163) -> (18.28, 8.163)
  line L4576 (18.78, 8.163) -> (19.78, 8.163)
  line L4577 (19.78, 8.163) -> (19.78, 9.163)
  line L4578 (19.78, 9.163) -> (18.78, 9.163)
  line L4579 (18.78, 9.163) -> (18.78, 8.163)
  line L4580 (19.28, 8.163) -> (20.28, 8.163)
  line L4581 (20.28, 8.163) -> (20.28, 9.163)
  line L4582 (20.28, 9.163) -> (19.28, 9.163)
  line L4583 (19.28, 9.163) -> (19.28, 8.163)
  line L4584 (19.78, 8.163) -> (20.78, 8.163)
  line L4585 (20.78, 8.163) -> (20.78, 9.163)
  line L4586 (20.78, 9.163) -> (19.78, 9.163)
  line L4587 (19.78, 9.163) -> (19.78, 8.163)
  line L4588 (20.28, 8.163) -> (21.28, 8.163)
  line L4589 (21.28, 8.163) -> (21.28, 9.163)
  line L4590 (21.28, 9.163) -> (20.28, 9.163)
  line L4591 (20.28, 9.163) -> (20.28, 8.163)
  line L4592 (20.78, 8.163) -> (21.78, 8.163)
  line L4593 (21.78, 8.163) -> (21.78, 9.163)
  line L4594 (21.78, 9.163) -> (20.78, 9.163)
  line L4595 (20.78, 9.163) -> (20.78, 8.163)
  line L4596 (21.28, 8.163) -> (22.28, 8.163)
  line L4597 (22.28, 8.163) -> (22.28, 9.163)
  line L4598 (22.28, 9.163) -> (21.28, 9.163)
  line L4599 (21.28, 9.163) -> (21.28, 8.163)
  line L4600 (21.78, 8.163) -> (22.78, 8.163)
  line L4601 (22.78, 8.163) -> (22.78, 9.163)
  line L4602 (22.78, 9.163) -> (21.78, 9.163)
  line L4603 (21.78, 9.163) -> (21.78, 8.163)
  line L4604 (22.28, 8.163) -> (23.28, 8.163)
  line L4605 (23.28, 8.163) -> (23.28, 9.163)
  line L4606 (23.28, 9.163) -> (22.28, 9.163)
  line L4607 (22.28, 9.163) -> (22.28, 8.163)
  line L4608 (22.78, 8.163) -> (23.78, 8.163)
  line L4609 (23.78, 8.163) -> (23.78, 9.163)
  line L4610 (23.78, 9.163) -> (22.78, 9.163)
  line L4611 (22.78, 9.163) -> (22.78, 8.163)
  line L4612 (23.28, 8.163) -> (24.28, 8.163)
  line L4613 (24.28, 8.163) -> (24.28, 9.163)
  line L4614 (24.28, 9.163) -> (23.28, 9.163)
  line L4615 (23.28, 9.163) -> (23.28, 8.163)
  line L4616 (25, 9.883) -> (26, 9.883)
  line L4617 (26, 9.883) -> (26, 10.883)
  line L4618 (26, 10.883) -> (25, 10.883)
  line L4619 (25, 10.883) -> (25, 9.883)
  line L4620 (25, 10.383) -> (26, 10.383)
  line L4621 (26, 10.383) -> (26, 11.383)
  line L4622 (26, 11.383) -> (25, 11.383)
  line L4623 (25, 11.383) -> (25, 10.383)
  line L4624 (25, 10.883) -> (26, 10.883)
  line L4625 (26, 10.883) -> (26, 11.883)
  line L4626 (26, 11.883) -> (25, 11.883)
  line L4627 (25, 11.883) -> (25, 10.883)
  line L4628 (25, 11.383) -> (26, 11.383)
  line L4629 (26, 11.383) -> (26, 12.383)
  line L4630 (26, 12.383) -> (25, 12.383)
  line L4631 (25, 12.383) -> (25, 11.383)
  line L4632 (25, 11.883) -> (26, 11.883)
  line L4633 (26, 11.883) -> (26, 12.883)
  line L4634 (26, 12.883) -> (25, 12.883)
  line L4635 (25, 12.883) -> (25, 11.883)
  line L4636 (25, 12.383) -> (26, 12.383)
  line L4637 (26, 12.383) -> (26, 13.383)
  line L4638 (26, 13.383) -> (25, 13.383)
  line L4639 (25, 13.383) -> (25, 12.383)
  line L4640 (25, 12.883) -> (26, 12.883)
  line L4641 (26, 12.883) -> (26, 13.883)
  line L4642 (26, 13.883) -> (25, 13.883)
  line L4643 (25, 13.883) -> (25, 12.883)
  line L4644 (25, 13.383) -> (26, 13.383)
  line L4645 (26, 13.383) -> (26, 14.383)
  line L4646 (26, 14.383) -> (25, 14.383)
  line L4647 (25, 14.383) -> (25, 13.383)
  line L4648 (25, 13.883) -> (26, 13.883)
  line L4649 (26, 13.883) -> (26, 14.883)
  line L4650 (26, 14.883) -> (25, 14.883)
  line L4651 (25, 14.883) -> (25, 13.883)
  line L4652 (25, 14.383) -> (26, 14.383)
  line L4653 (26, 14.383) -> (26, 15.383)
  line L4654 (26, 15.383) -> (25, 15.383)
  line L4655 (25, 15.383) -> (25, 14.383)
  line L4656 (25, 14.883) -> (26, 14.883)
  line L4657 (26, 14.883) -> (26, 15.883)
  line L4658 (26, 15.883) -> (25, 15.883)
  line L4659 (25, 15.883) -> (25, 14.883)
  line L4660 (25, 15.383) -> (26, 15.383)
  line L4661 (26, 15.383) -> (26, 16.383)
  line L4662 (26, 16.383) -> (25, 16.383)
  line L4663 (25, 16.383) -> (25, 15.383)
  line L4664 (25, 15.883) -> (26, 15.883)
  line L4665 (26, 15.883) -> (26, 16.883)
  line L4666 (26, 16.883) -> (25, 16.883)
  line L4667 (25, 16.883) -> (25, 15.883)
  line L4668 (25, 16.383) -> (26, 16.383)
  line L4669 (26, 16.383) -> (26, 17.383)
  line L4670 (26, 17.383) -> (25, 17.383)
  line L4671 (25, 17.383) -> (25, 16.383)
  line L4672 (25, 16.883) -> (26, 16.883)
  line L4673 (26, 16.883) -> (26, 17.883)
  line L4674 (26, 17.883) -> (25, 17.883)
  line L4675 (25, 17.883) -> (25, 16.883)
  line L4676 (25, 17.383) -> (26, 17.383)
  line L4677 (26, 17.383) -> (26, 18.383)
  line L4678 (26, 18.383) -> (25, 18.383)
  line L4679 (25, 18.383) -> (25, 17.383)
  line L4680 (25, 17.883) -> (26, 17.883)
  line L4681 (26, 17.883) -> (26, 18.883)
  line L4682 (26, 18.883) -> (25, 18.883)
  line L4683 (25, 18.883) -> (25, 17.883)
  line L4684 (25, 18.383) -> (26, 18.383)
  line L4685 (26, 18.383) -> (26, 19.383)
  line L4686 (26, 19.383) -> (25, 19.383)
  line L4687 (25, 19.383) -> (25, 18.383)
  line L4688 (25, 18.883) -> (26, 18.883)
  line L4689 (26, 18.883) -> (26, 19.883)
  line L4690 (26, 19.883) -> (25, 19.883)
  line L4691 (25, 19.883) -> (25, 18.883)
  line L4692 (25, 19.383) -> (26, 19.383)
  line L4693 (26, 19.383) -> (26, 20.383)
  line L4694 (26, 20.383) -> (25, 20.383)
  line L4695 (25, 20.383) -> (25, 19.383)
  line L4696 (25, 19.883) -> (26, 19.883)
  line L4697 (26, 19.883) -> (26, 20.883)
  line L4698 (26, 20.883) -> (25, 20.883)
  line L4699 (25, 20.883) -> (25, 19.883)
  line L4700 (25, 20.383) -> (26, 20.383)
  line L4701 (26, 20.383) -> (26, 21.383)
  line L4702 (26, 21.383) -> (25, 21.383)
  line L4703 (25, 21.383) -> (25, 20.383)
  line L4704 (25, 20.883) -> (26, 20.883)
  line L4705 (26, 20.883) -> (26, 21.883)
  line L4706 (26, 21.883) -> (25, 21.883)
  line L4707 (25, 21.883) -> (25, 20.883)
  line L4708 (25, 21.383) -> (26, 21.383)
  line L4709 (26, 21.383) -> (26, 22.383)
  line L4710 (26, 22.383) -> (25, 22.383)
  line L4711 (25, 22.383) -> (25, 21.383)
  line L4712 (25, 21.883) -> (26, 21.883)
  line L4713 (26, 21.883) -> (26, 22.883)
  line L4714 (26, 22.883) -> (25, 22.883)
  line L4715 (25, 22.883) -> (25, 21.883)
  line L4716 (23.28, 23.603) -> (24.28, 23.603)
  line L4717 (24.28, 23.603) -> (24.28, 24.603)
  line L4718 (24.28, 24.603) -> (23.28, 24.603)
  line L4719 (23.28, 24.603) -> (23.28, 23.603)
  line L4720 (22.78, 23.603) -> (23.78, 23.603)
  line L4721 (23.78, 23.603) -> (23.78, 24.603)
  line L4722 (23.78, 24.603) -> (22.78, 24.603)
  line L4723 (22.78, 24.603) -> (22.78, 23.603)
  line L4724 (22.28, 23.603) -> (23.28, 23.603)
  line L4725 (23.28, 23.603) -> (23.28, 24.603)
  line L4726 (23.28, 24.603) -> (22.28, 24.603)
  line L4727 (22.28, 24.603) -> (22.28, 23.603)
  line L4728 (21.78, 23.603) -> (22.78, 23.603)
  line L4729 (22.78, 23.603) -> (22.78, 24.603)
  line L4730 (22.78, 24.603) -> (21.78, 24.603)
  line L4731 (21.78, 24.603) -> (21.78, 23.603)
  line L4732 (21.28, 23.603) -> (22.28, 23.603)
  line L4733 (22.28, 23.603) -> (22.28, 24.603)
  line L4734 (22.28, 24.603) -> (21.28, 24.603)
  line L4735 (21.28, 24.603) -> (21.28, 23.603)
  line L4736 (20.78, 23.603) -> (21.78, 23.603)
  line L4737 (21.78, 23.603) -> (21.78, 24.603)
  line L4738 (21.78, 24.603) -> (20.78, 24.603)
  line L4739 (20.78, 24.603) -> (20.78, 23.603)
  line L4740 (20.28, 23.603) -> (21.28, 23.603)
  line L4741 (21.28, 23.603) -> (21.28, 24.603)
  line L4742 (21.28, 24.603) -> (20.28, 24.603)
  line L4743 (20.28, 24.603) -> (20.28, 23.603)
  line L4744 (19.78, 23.603) -> (20.78, 23.603)
  line L4745 (20.78, 23.603) -> (20.78, 24.603)
  line L4746 (20.78, 24.603) -> (19.78, 24.603)
  line L4747 (19.78, 24.603) -> (19.78, 23.603)
  line L4748 (19.28, 23.603) -> (20.28, 23.603)
  line L4749 (20.28, 23.603) -> (20.28, 24.603)
  line L4750 (20.28, 24.603) -> (19.28, 24.603)
  line L4751 (19.28, 24.603) -> (19.28, 23.603)
  line L4752 (18.78, 23.603) -> (19.78, 23.603)
  line L4753 (19.78, 23.603) -> (19.78, 24.603)
  line L4754 (19.78, 24.603) -> (18.78, 24.603)
  line L4755 (18.78, 24.603) -> (18.78, 23.603)
  line L4756 (18.28, 23.603) -> (19.28, 23.603)
  line L4757 (19.28, 23.603) -> (19.28, 24.603)
  line L4758 (19.28, 24.603) -> (18.28, 24.603)
  line L4759 (18.28, 24.603) -> (18.28, 23.603)
  line L4760 (17.78, 23.603) -> (18.78, 23.603)
  line L4761 (18.78, 23.603) -> (18.78, 24.603)
  line L4762 (18.78, 24.603) -> (17.78, 24.603)
  line L4763 (17.78, 24.603) -> (17.78, 23.603)
  line L4764 (17.28, 23.603) -> (18.28, 23.603)
  line L4765 (18.28, 23.603) -> (18.28, 24.603)
  line L4766 (18.28, 24.603) -> (17.28, 24.603)
  line L4767 (17.28, 24.603) -> (17.28, 23.603)
  line L4768 (16.78, 23.603) -> (17.78, 23.603)
  line L4769 (17.78, 23.603) -> (17.78, 24.603)
  line L4770 (17.78, 24.603) -> (16.78, 24.603)
  line L4771 (16.78, 24.603) -> (16.78, 23.603)
  line L4772 (16.28, 23.603) -> (17.28, 23.603)
  line L4773 (17.28, 23.603) -> (17.28, 24.603)